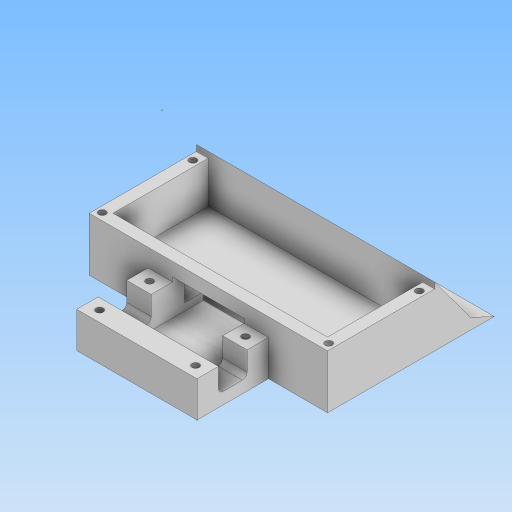
# Autodesk Inventor part: MINISUMO_BODY_V2
Saved by Autodesk Inventor 2023.2 (Build 272271000, 271)
## iProperties
Created: 2023-01-25
Part Number: MINISUMO_BODY_V2
Material: Generic
Document SubType Name: Modeling
Designer: MenMe
Density: 1 g/cm^3
Appearance: Default
Author: MenMe
Autodesk Inventor part; units mm, degrees
ref_plane "YZ Plane" through (0, 0, 0) normal (1, 0, 0) x (0, 1, 0)
ref_plane "XZ Plane" through (0, 0, 0) normal (0, 1, 0) x (-1, 0, 0)
ref_plane "XY Plane" through (0, 0, 0) normal (0, 0, 1) x (1, 0, 0)
sketch "Sketch2" plane through (0, 0, 0) normal (1, 0, 0) x (0, 1, 0)
  line L0 (0, -30) -> (0, -100)
  line L1 (22.5, -30) -> (0, -30)
  line L2 (0, -100) -> (4.6583, -90)
  line L3 (4.6583, -90) -> (25, -75)
  line L4 (25, -75) -> (5, -75)
  line L5 (5, -75) -> (5, -35)
  line L6 (5, -35) -> (22.5, -35)
  line L7 (22.5, -35) -> (22.5, -30)
  line L8 (5, -75) -> (22.5, -75)
  line L9 (22.5, -35) -> (5, -35)
  line L10 (5, -35) -> (5, -75)
  point P0 (0, 0)
  dimension "d0" = 100
  dimension "d3" = 22.5
  dimension "d23" = 5
  dimension "d24" = 5
  dimension "d25" = 40
  dimension "d26" = 10
  dimension "d27" = 70
  dimension "d60" = 25
  constraints: 22 end point, 4 perpendicular, 2 horizontal, 1 parallel
  measures "d0" distance of L0.end point (0, 0)
  measures "d3" distance of L1.start L0.start
  measures "d23" distance between parallel lines of L0 L5
  measures "d24" distance between parallel lines of L1 L6
  measures "d25" distance of L4.end L5.end
  measures "d26" vertical distance of L0.end L2.end
  measures "d27" distance of L0.end L0.start
  measures "d60" distance from line of L0 L3.end
extrude "Extrusion1" add sketch "Sketch2" along normal blind 100
sketch "Sketch5" plane through (0, 0, -100) normal (0, -1, 0) x (1, 0, 0)
  line L0 (0, 70) -> (100, 70) projected
  line L1 (75.25, 70) -> (24.75, 70)
  line L2 (24.75, 70) -> (24.75, 100)
  line L3 (24.75, 100) -> (75.25, 100)
  line L4 (75.25, 100) -> (75.25, 70)
  point P0 (0, 100)
  point P1 (24.75, 70)
  dimension "d19" = 30
  dimension "d20" = 24.75
  dimension "d21" = 24.75
  dimension "d22" = 50.5
  constraints: 8 end point, 2 parallel, 1 horizontal, 1 perpendicular, 1 point on line
  measures "d19" distance of L1.end L2.end
  measures "d20" distance from line of L0.end L4
  measures "d21" distance from line of L0.start L2
  measures "d22" distance of L2.end L3.end
extrude "Extrusion3" add sketch "Sketch5" against normal blind 20
sketch "Sketch6" plane through (75.25, 0, 0) normal (1, 0, 0) x (0, 0, -1)
  point P0 (0, 0)
sketch "Sketch7" plane through (75.25, 0, 0) normal (1, 0, 0) x (0, 0, -1)
  point P0 (0, 0)
sketch "Sketch8" plane through (75.25, 0, 0) normal (1, 0, 0) x (0, 0, -1)
  line L0 (9, 15) -> (21, 15)
  line L1 (21, 15) -> (21, 5)
  line L2 (21, 5) -> (9, 5)
  line L3 (9, 5) -> (9, 15)
  line L4 (30, 22.5) -> (30, 0) projected
  line L5 (0, 20) -> (30, 20) projected
  point P0 (0, 0)
  point P1 (15.1042, 20)
  dimension "d30" = 12
  dimension "d31" = 10
  dimension "d32" = 9
  dimension "d33" = 5
  constraints: 8 end point, 2 parallel, 1 horizontal, 1 perpendicular, 2 other
  measures "d30" distance of L1.end L2.end
  measures "d31" distance of L0.end L1.end
  measures "d32" distance between parallel lines of L4 L1
  measures "d33" distance from line of point (15.104, 20) L0
extrude "Extrusion4" cut sketch "Sketch8" against normal through all
fillet "Fillet1" radius 2 4 edges at (50, 5, -9) (50, 15, -21) (50, 15, -9) (50, 5, -21)
sketch "Sketch9" plane through (75.25, 0, 0) normal (1, 0, 0) x (0, 0, -1)
  arc A0 (11, 15) -> (9, 13) centre (11, 13) ccw projected
  line L0 (11, 15) -> (0, 15)
  arc A1 (21, 13) -> (19, 15) centre (19, 13) ccw projected
  line L1 (19, 15) -> (30, 15)
  line L2 (30, 0) -> (30, 20) projected
  line L3 (30, 20) -> (0, 20) projected
  line L4 (0, 20) -> (30, 20)
  line L5 (30, 20) -> (30, 15)
  line L6 (30, 15) -> (0, 15)
  line L7 (0, 15) -> (0, 20)
  point P0 (0, 0)
  point P1 (0, 15)
  point P2 (11, 15)
  point P3 (19, 15)
  constraints: 12 end point, 3 horizontal, 2 parallel, 1 perpendicular, 1 point on circle, 1 point on line, 1 tangent
extrude "Extrusion5" cut sketch "Sketch9" against normal through all
sketch "Sketch10" plane through (75.25, 0, 0) normal (1, 0, 0) x (0, 0, -1)
  arc A0 (11, 15) -> (9, 13) centre (11, 13) ccw projected
  line L0 (9, 13) -> (9, 15)
  line L1 (9, 15) -> (11, 15)
  point P0 (0, 0)
  constraints: 4 end point, 2 tangent, 1 perpendicular, 1 vertical
extrude "Extrusion6" cut sketch "Sketch10" against normal through all
sketch "Sketch11" plane through (75.25, 0, 0) normal (1, 0, 0) x (0, 0, -1)
  arc A0 (21, 13) -> (19, 15) centre (19, 13) ccw projected
  line L0 (21, 13) -> (21, 15)
  line L1 (19, 15) -> (30, 15) projected
  line L2 (21, 15) -> (19, 15)
  point P0 (0, 0)
  constraints: 4 end point, 1 collinear, 1 tangent, 1 vertical
extrude "Extrusion7" cut sketch "Sketch11" against normal through all
sketch "Sketch13" plane through (0, 5, -35) normal (0, 0, -1) x (-1, 0, 0)
  line L0 (-65, 11.888) -> (-35, 11.888)
  line L1 (-35, 11.888) -> (-35, -3.112)
  line L2 (-35, -3.112) -> (-65, -3.112)
  line L3 (-65, -3.112) -> (-65, 11.888)
  line L4 (0, 0) -> (0, 17.5) projected
  point P0 (0, -5)
  dimension "d43" = 15
  dimension "d44" = 30
  dimension "d45" = 35
  constraints: 8 end point, 2 parallel, 1 horizontal, 1 perpendicular
  measures "d43" distance of L0.end L1.end
  measures "d44" distance of L0.end L0.start
  measures "d45" distance between parallel lines of L4 L1
extrude "Extrusion8" cut sketch "Sketch13" along normal blind 8 and the other way blind 20
sketch "Sketch18" plane through (0, 4.6583, -90) normal (0, 0.9064745, -0.4222605) x (1, 0, 0)
  line L0 (59.644, 5.17) -> (-2.9092, 5.17) construction
  line L1 (-2.9092, 5.17) -> (-2.9092, 12.9891) construction
  line L2 (-2.9092, 12.9891) -> (59.644, 12.9891) construction
  line L3 (59.644, 12.9891) -> (59.644, 5.17) construction
  spline S0 degree 2 poles (58.4033, 8.3337) (58.7542, 8.3337) (59.2387, 8.1977) (59.4315, 8.0989) knots 0 0 0 1 2 2 2
  line L4 (59.4315, 8.0989) -> (59.1843, 7.3722)
  line L5 (59.1843, 7.3722) -> (59.1151, 7.3722)
  spline S1 degree 2 poles (59.1151, 7.3722) (58.952, 7.5675) (58.4725, 7.7776) (58.213, 7.7776) knots 0 0 0 1 2 2 2
  spline S2 degree 2 poles (58.213, 7.7776) (58.1462, 7.7776) (57.9213, 7.7479) (57.8472, 7.7182) knots 0 0 0 1 2 2 2
  spline S3 degree 2 poles (57.8472, 7.7182) (57.7557, 7.6836) (57.6025, 7.5576) (57.5679, 7.4562) knots 0 0 0 1 2 2 2
  spline S4 degree 2 poles (57.5679, 7.4562) (57.5283, 7.3401) (57.6593, 7.1967) (57.773, 7.1646) knots 0 0 0 1 2 2 2
  spline S5 degree 2 poles (57.773, 7.1646) (57.9139, 7.1226) (58.2426, 7.0509) (58.3786, 6.9965) knots 0 0 0 1 2 2 2
  spline S6 degree 2 poles (58.3786, 6.9965) (58.69, 6.8729) (58.8556, 6.4503) (58.7468, 6.1339) knots 0 0 0 1 2 2 2
  spline S7 degree 2 poles (58.7468, 6.1339) (58.601, 5.7063) (57.6964, 5.1749) (57.1526, 5.1749) knots 0 0 0 1 2 2 2
  spline S8 degree 2 poles (57.1526, 5.1749) (56.8807, 5.1749) (56.3815, 5.2861) (56.1986, 5.3801) knots 0 0 0 1 2 2 2
  line L6 (56.1986, 5.3801) -> (56.4359, 6.0771)
  line L7 (56.4359, 6.0771) -> (56.5051, 6.0771)
  spline S9 degree 2 poles (56.5051, 6.0771) (56.6237, 5.9312) (57.0439, 5.731) (57.3034, 5.731) knots 0 0 0 1 2 2 2
  spline S10 degree 2 poles (57.3034, 5.731) (57.4023, 5.731) (57.5728, 5.7607) (57.6741, 5.8002) knots 0 0 0 1 2 2 2
  spline S11 degree 2 poles (57.6741, 5.8002) (57.7557, 5.8324) (57.904, 5.9609) (57.9312, 6.04) knots 0 0 0 1 2 2 2
  spline S12 degree 2 poles (57.9312, 6.04) (57.9707, 6.1586) (57.8521, 6.2946) (57.6346, 6.3489) knots 0 0 0 1 2 2 2
  spline S13 degree 2 poles (57.6346, 6.3489) (57.4912, 6.3836) (57.2292, 6.4503) (57.0884, 6.5071) knots 0 0 0 1 2 2 2
  spline S14 degree 2 poles (57.0884, 6.5071) (56.8091, 6.6233) (56.6311, 7.0089) (56.7399, 7.3252) knots 0 0 0 1 2 2 2
  spline S15 degree 2 poles (56.7399, 7.3252) (56.8931, 7.78) (57.7953, 8.3337) (58.4033, 8.3337) knots 0 0 0 1 2 2 2
  spline S16 degree 2 poles (54.2312, 8.3436) (54.8466, 8.3436) (55.3063, 7.7504) (55.1135, 7.1769) knots 0 0 0 1 2 2 2
  line L8 (55.1135, 7.1769) -> (54.4511, 5.2293)
  line L9 (54.4511, 5.2293) -> (53.6849, 5.2293)
  line L10 (53.6849, 5.2293) -> (54.33, 7.1325)
  spline S17 degree 2 poles (54.33, 7.1325) (54.4388, 7.4513) (54.3053, 7.7627) (54.0334, 7.7627) knots 0 0 0 1 2 2 2
  spline S18 degree 2 poles (54.0334, 7.7627) (53.769, 7.7627) (53.4205, 7.4637) (53.3068, 7.1325) knots 0 0 0 1 2 2 2
  line L11 (53.3068, 7.1325) -> (52.6617, 5.2293)
  line L12 (52.6617, 5.2293) -> (51.8955, 5.2293)
  line L13 (51.8955, 5.2293) -> (52.5554, 7.1745)
  spline S19 degree 2 poles (52.5554, 7.1745) (52.7482, 7.738) (53.5984, 8.3436) (54.2312, 8.3436) knots 0 0 0 1 2 2 2
  line L14 (48.0002, 8.2793) -> (48.7614, 8.2793)
  line L15 (48.7614, 8.2793) -> (48.0743, 6.2575)
  line L16 (48.0743, 6.2575) -> (49.0728, 7.5625)
  line L17 (49.0728, 7.5625) -> (49.5944, 7.5625)
  line L18 (49.5944, 7.5625) -> (49.7056, 6.2575)
  line L19 (49.7056, 6.2575) -> (50.3927, 8.2793)
  line L20 (50.3927, 8.2793) -> (51.1144, 8.2793)
  line L21 (51.1144, 8.2793) -> (50.0788, 5.2293)
  line L22 (50.0788, 5.2293) -> (49.194, 5.2293)
  line L23 (49.194, 5.2293) -> (49.0308, 6.7345)
  line L24 (49.0308, 6.7345) -> (47.8444, 5.2293)
  line L25 (47.8444, 5.2293) -> (46.9645, 5.2293)
  line L26 (46.9645, 5.2293) -> (48.0002, 8.2793)
  line L27 (46.139, 8.2793) -> (45.1034, 5.2293)
  line L28 (45.1034, 5.2293) -> (43.0421, 5.2293)
  line L29 (43.0421, 5.2293) -> (43.2373, 5.8101)
  line L30 (43.2373, 5.8101) -> (44.5374, 5.8101)
  line L31 (44.5374, 5.8101) -> (44.7203, 6.3465)
  line L32 (44.7203, 6.3465) -> (43.5215, 6.3465)
  line L33 (43.5215, 6.3465) -> (43.7193, 6.9273)
  line L34 (43.7193, 6.9273) -> (44.918, 6.9273)
  line L35 (44.918, 6.9273) -> (45.18, 7.6985)
  line L36 (45.18, 7.6985) -> (43.8799, 7.6985)
  line L37 (43.8799, 7.6985) -> (44.0777, 8.2793)
  line L38 (44.0777, 8.2793) -> (46.139, 8.2793)
  spline S20 degree 2 poles (41.0351, 8.3386) (41.7222, 8.3386) (42.2462, 7.5081) (41.9916, 6.7568) knots 0 0 0 1 2 2 2
  spline S21 degree 2 poles (41.9916, 6.7568) (41.7444, 6.0326) (40.6421, 5.17) (39.9574, 5.17) knots 0 0 0 1 2 2 2
  spline S22 degree 2 poles (39.9574, 5.17) (39.7745, 5.17) (39.4977, 5.212) (39.3766, 5.2466) knots 0 0 0 1 2 2 2
  spline S23 degree 2 poles (39.3766, 5.2466) (39.2827, 5.2787) (39.0751, 5.385) (39.0108, 5.4246) knots 0 0 0 1 2 2 2
  line L39 (39.0108, 5.4246) -> (39.258, 6.1512)
  line L40 (39.258, 6.1512) -> (39.3371, 6.1512)
  spline S24 degree 2 poles (39.3371, 6.1512) (39.3741, 6.1018) (39.4953, 5.9634) (39.5793, 5.8991) knots 0 0 0 1 2 2 2
  spline S25 degree 2 poles (39.5793, 5.8991) (39.6633, 5.8324) (39.8882, 5.7409) (40.0291, 5.7409) knots 0 0 0 1 2 2 2
  spline S26 degree 2 poles (40.0291, 5.7409) (40.1947, 5.7409) (40.5062, 5.8447) (40.6742, 5.9757) knots 0 0 0 1 2 2 2
  spline S27 degree 2 poles (40.6742, 5.9757) (40.8275, 6.0919) (41.1092, 6.4898) (41.2007, 6.7592) knots 0 0 0 1 2 2 2
  spline S28 degree 2 poles (41.2007, 6.7592) (41.2971, 7.0435) (41.2773, 7.4315) (41.1957, 7.5502) knots 0 0 0 1 2 2 2
  spline S29 degree 2 poles (41.1957, 7.5502) (41.1166, 7.6663) (40.8571, 7.7677) (40.7138, 7.7677) knots 0 0 0 1 2 2 2
  spline S30 degree 2 poles (40.7138, 7.7677) (40.5605, 7.7677) (40.254, 7.6663) (40.1379, 7.6045) knots 0 0 0 1 2 2 2
  spline S31 degree 2 poles (40.1379, 7.6045) (40.0143, 7.5428) (39.8141, 7.4118) (39.7399, 7.3598) knots 0 0 0 1 2 2 2
  line L41 (39.7399, 7.3598) -> (39.6707, 7.3598)
  line L42 (39.6707, 7.3598) -> (39.913, 8.0766)
  spline S32 degree 2 poles (39.913, 8.0766) (40.0094, 8.1162) (40.2664, 8.215) (40.3949, 8.2496) knots 0 0 0 1 2 2 2
  spline S33 degree 2 poles (40.3949, 8.2496) (40.5531, 8.2941) (40.8176, 8.3386) (41.0351, 8.3386) knots 0 0 0 1 2 2 2
  point P0 (0, -79.6157)
  constraints: 2 other
extrude "Extrusion11" cut sketch "Sketch18" against normal through all
sketch "Sketch25" plane through (75.25, 15, 0) normal (0, 1, 0) x (1, 0, 0)
  circle A0 centre (-45.375, 4.5) radius 1.5
  circle A1 centre (-5.125, 4.5) radius 1.5
  circle A2 centre (-5.125, 25.5) radius 1.5
  circle A3 centre (-45.375, 25.5) radius 1.5
  line L0 (-50.5, 21) -> (-50.5, 30) projected
  line L1 (-50.5, 0) -> (-50.5, 9) projected
  line L2 (0, 9) -> (0, 0) projected
  line L3 (0, 30) -> (0, 21) projected
  line L4 (-75.25, 30) -> (24.75, 30) projected
  line L5 (0, 9) -> (-50.5, 9) projected
  point P0 (-75.25, 0)
  point P1 (-50.5, 4.5)
  point P2 (0, 25.5)
  dimension "d63" = 3
  dimension "d64" = 5.125
  dimension "d65" = 5.125
  dimension "d66" = 5.125
  dimension "d67" = 5.125
  dimension "d89" = 4.5
  dimension "d90" = 4.5
  dimension "d91" = 4.5
  dimension "d92" = 4.5
  constraints: 4 centre point, 3 equal radius, 2 midpoint
  measures "d63" diameter of A0
  measures "d64" distance from line of L0 A3.centre
  measures "d65" distance of point (-50.5, 4.5) A0.centre
  measures "d66" distance from line of L2 A1.centre
  measures "d67" distance of A2.centre point (0, 25.5)
  measures "d89" distance from line of L4 A3.centre
  measures "d90" distance from line of L4 A2.centre
  measures "d91" distance from line of L5 A0.centre
  measures "d92" distance from line of L5 A1.centre
extrude "Extrusion12" cut sketch "Sketch25" against normal blind 10
sketch "Sketch28" plane through (0, 22.5, -30) normal (0, 1, 0) x (1, 0, 0)
  circle A0 centre (2.5, 41) radius 1.5
  circle A1 centre (2.5, 3) radius 1.5
  circle A2 centre (97.5, 41) radius 1.5
  circle A3 centre (97.5, 3) radius 1.5
  line L0 (100, 45) -> (100, 0) projected
  line L1 (0, 45) -> (100, 45) projected
  line L2 (5, 45) -> (5, 5) projected
  line L3 (0, 45) -> (100, 45) projected
  line L4 (0, 0) -> (100, 0) projected
  point P0 (0, -30)
  point P1 (95, 45)
  point P2 (2.5, 45)
  dimension "d75" = 3
  dimension "d76" = 2.5
  dimension "d77" = 3
  dimension "d78" = 2.5
  dimension "d79" = 4
  dimension "d80" = 2.5
  dimension "d81" = 4
  dimension "d82" = 2.5
  dimension "d83" = 3
  dimension "d84" = 3
  constraints: 4 centre point, 2 equal radius, 1 point on line
  measures "d75" diameter of A0
  measures "d76" distance from line of L0 A2.centre
  measures "d77" diameter of A2
  measures "d78" distance from line of L0 A3.centre
  measures "d79" distance from line of L1 A2.centre
  measures "d80" distance from line of L2 A0.centre
  measures "d81" distance of point (2.5, 45) A0.centre
  measures "d82" distance from line of L2 A1.centre
  measures "d83" distance from line of L4 A1.centre
  measures "d84" distance from line of L4 A3.centre
sketch "Sketch29" plane through (0, 0, 0) normal (-1, 0, 0) x (0, 0, 1)
  line L0 (-75, 25) -> (-75, 5) projected
  line L1 (-35, 5) -> (-35, 22.5) projected
  line L2 (-75, 5) -> (-35, 5)
  line L3 (-35, 5) -> (-35, 22.5)
  line L4 (-35, 22.5) -> (-75, 22.5)
  line L5 (-75, 22.5) -> (-75, 5)
  line L6 (-75, 5) -> (-35, 5)
  line L7 (-35, 5) -> (-35, 22.5)
  line L8 (-35, 22.5) -> (-75, 22.5)
  line L9 (-75, 22.5) -> (-75, 5)
  point P0 (0, 0)
  constraints: 16 end point, 4 parallel, 2 horizontal, 2 perpendicular
extrude "Extrusion15" add sketch "Sketch29" against normal blind 5
sketch "Sketch30" plane through (100, 0, 0) normal (1, 0, 0) x (0, 0, -1)
  line L0 (75, 5) -> (35, 5) projected
  line L1 (35, 5) -> (35, 22.5) projected
  line L2 (75, 5) -> (35, 5)
  line L3 (35, 5) -> (35, 22.5)
  line L4 (35, 22.5) -> (75, 22.5)
  line L5 (75, 22.5) -> (75, 5)
  point P0 (0, 0)
  constraints: 8 end point, 2 parallel, 1 horizontal, 1 perpendicular
extrude "Extrusion16" add sketch "Sketch30" against normal blind 5
thread "Thread1" size "M3x0.5" class "6H" standard "ANSI Metric M Profile" full length
thread "Thread2" size "M3x0.5" class "6H" standard "ANSI Metric M Profile" full length
thread "Thread3" size "M3x0.5" class "6H" standard "ANSI Metric M Profile" full length
thread "Thread4" size "M3x0.5" class "6H" standard "ANSI Metric M Profile" full length
extrude "Extrusion17" cut sketch "Sketch28" against normal blind 10
thread "Thread5" size "M3x0.5" class "6H" standard "ANSI Metric M Profile" full length
thread "Thread6" size "M3x0.5" class "6H" standard "ANSI Metric M Profile" full length
thread "Thread7" size "M3x0.5" class "6H" standard "ANSI Metric M Profile" full length
thread "Thread8" size "M3x0.5" class "6H" standard "ANSI Metric M Profile" full length
sketch "Sketch31" plane through (100, 25, -75) normal (0, 0.5934903, -0.8048412) x (-1, 0, 0)
  point P0 (100, 24.3907)
sketch "Sketch32" plane through (100, 25, -75) normal (0, 0.5934903, -0.8048412) x (-1, 0, 0)
  point P0 (100, 24.3907)
sketch "Sketch33" plane through (100, 25, -75) normal (0, 0.5934903, -0.8048412) x (-1, 0, 0)
  point P0 (100, 24.3907)
body "Solid1"
